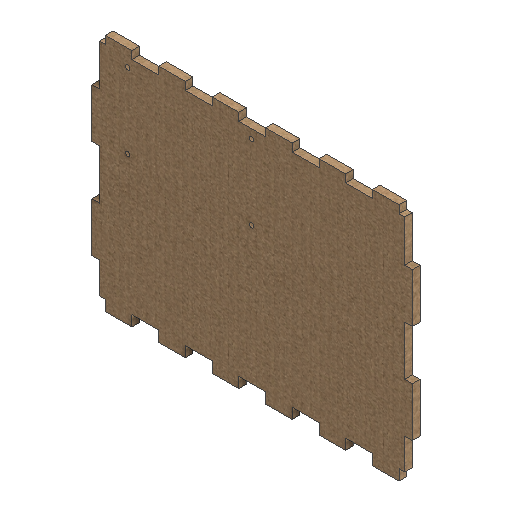
# Autodesk Inventor part: FloorPlate_1
Saved by Autodesk Inventor 2025.2 (Build 292293000, 293)
## iProperties
Created: 2025-03-07
Part Number: FloorPlate_1
Material: MDF Medium Density Fiberboard
Document SubType Name: Modeling
Designer: ahorat
Density: 0.8 g/cm^3
Appearance: Cardboard - Corrugated
Author: ahorat
Autodesk Inventor part; units mm, degrees
ref_plane "YZ Plane" through (0, 0, 0) normal (1, 0, 0) x (0, 1, 0)
ref_plane "XZ Plane" through (0, 0, 0) normal (0, 1, 0) x (-1, 0, 0)
ref_plane "XY Plane" through (0, 0, 0) normal (0, 0, 1) x (1, 0, 0)
sketch "Sketch1" plane through (0, 0, 0) normal (0, 0, 1) x (1, 0, 0)
  line L0 (-105, -80.9) -> (105, -80.9)
  line L1 (105, -80.9) -> (105, 80.9)
  line L2 (105, 80.9) -> (-105, 80.9)
  line L3 (-105, 80.9) -> (-105, -80.9)
  line L4 (-105, -80.9) -> (105, 80.9) construction
  line L5 (105, -80.9) -> (-105, 80.9) construction
  point P0 (0, 0)
  dimension "d0" = 210
  dimension "d1" = 161.8
  constraints: 12 end point, 2 midpoint, 2 parallel, 1 horizontal, 1 perpendicular
  measures "d0" distance of L1.end L2.end
  measures "d1" distance of L0.end L1.end
extrude "Extrusion1" add sketch "Sketch1" along normal blind 5
sketch "Sketch3" plane through (0, 0, 0) normal (0, 0, -1) x (-1, 0, 0)
  line L0 (0.5, 69.9) -> (81.5, 69.9)
  line L1 (81.5, 69.9) -> (81.5, 20.9)
  line L2 (81.5, 20.9) -> (0.5, 20.9)
  line L3 (0.5, 20.9) -> (0.5, 69.9)
  line L4 (105, 80.9) -> (105, -80.9) projected
  line L5 (-105, 80.9) -> (105, 80.9) projected
  point P0 (0, 0)
  dimension "d20" = 49
  dimension "d21" = 81
  dimension "d22" = 23.5
  dimension "d23" = 11
  constraints: 8 end point, 4 coincident, 2 parallel, 1 horizontal, 1 perpendicular
  measures "d20" distance of L2.end L0.start
  measures "d21" distance of L0.start L0.end
  measures "d22" distance between parallel lines of L4 L1
  measures "d23" distance between parallel lines of L5 L0
hole "Hole2" at (-0.5, 69.9, 0) at (-81.5, 69.9, 0) at (-0.5, 20.9, 0) at (-81.5, 20.9, 0) direction (0, 0, 1) diameter 3 end through all countersink diameter 4 countersink angle 90
sketch "Sketch4" plane through (0, 0, 0) normal (0, 0, -1) x (-1, 0, 0)
  line L0 (-105, 80.9) -> (105, 80.9) projected
  circle A0 centre (81.5, 20.9) radius 2 projected
  circle A1 centre (0.5, 20.9) radius 2 projected
  circle A2 centre (81.5, 69.9) radius 2 projected
  circle A3 centre (0.5, 69.9) radius 2 projected
  line L1 (-105, -80.9) -> (-105, 80.9) projected
  line L2 (105, -80.9) -> (-105, -80.9) projected
  line L3 (105, 80.9) -> (105, -80.9) projected
  line L4 (-105, 80.9) -> (105, 80.9) projected
  line L5 (8.8, 80.9) -> (-8.8, 80.9)
  line L6 (-8.8, 80.9) -> (-8.8, 75.8)
  line L7 (-8.8, 75.8) -> (8.8, 75.8)
  line L8 (8.8, 75.8) -> (8.8, 80.9)
  line L9 (-26.2, 75.8) -> (-26.2, 80.9)
  line L10 (-26.2, 80.9) -> (-43.8, 80.9)
  line L11 (-43.8, 80.9) -> (-43.8, 75.8)
  line L12 (-43.8, 75.8) -> (-26.2, 75.8)
  line L13 (-61.2, 75.8) -> (-61.2, 80.9)
  line L14 (-61.2, 80.9) -> (-78.8, 80.9)
  line L15 (-78.8, 80.9) -> (-78.8, 75.8)
  line L16 (-78.8, 75.8) -> (-61.2, 75.8)
  line L17 (-96.2, 75.8) -> (-96.2, 80.9)
  line L18 (-96.2, 80.9) -> (-113.8, 80.9)
  line L19 (-113.8, 80.9) -> (-113.8, 75.8)
  line L20 (-113.8, 75.8) -> (-96.2, 75.8)
  line L21 (26.2, 80.9) -> (26.2, 75.8)
  line L22 (43.8, 80.9) -> (26.2, 80.9)
  line L23 (43.8, 75.8) -> (43.8, 80.9)
  line L24 (26.2, 75.8) -> (43.8, 75.8)
  line L25 (61.2, 80.9) -> (61.2, 75.8)
  line L26 (78.8, 80.9) -> (61.2, 80.9)
  line L27 (78.8, 75.8) -> (78.8, 80.9)
  line L28 (61.2, 75.8) -> (78.8, 75.8)
  line L29 (96.2, 80.9) -> (96.2, 75.8)
  line L30 (113.8, 80.9) -> (96.2, 80.9)
  line L31 (113.8, 75.8) -> (113.8, 80.9)
  line L32 (96.2, 75.8) -> (113.8, 75.8)
  line L33 (0, 0) -> (105, 0) construction
  point P0 (0, 75.8)
  point P1 (8.8, 80.9)
  point P2 (-8.8, 80.9)
  point P3 (0, 80.9)
  point P4 (-35, 80.9)
  point P5 (-35, 75.8)
  point P6 (-70, 80.9)
  point P7 (-70, 75.8)
  point P8 (-105, 80.9)
  point P9 (-105, 75.8)
  point P10 (35, 75.8)
  point P11 (35, 80.9)
  point P12 (70, 75.8)
  point P13 (70, 80.9)
  point P14 (105, 75.8)
  point P15 (105, 80.9)
  point P16 (-105, 75.8)
  point P17 (105, 75.8)
  dimension "d43" = 210
  dimension "d44" = 17.6
  dimension "d45" = 5.1
  dimension "d48" = 35
  dimension "d55" = 35
  constraints: 58 end point, 3 horizontal, 3 midpoint, 2 parallel, 1 perpendicular, 1 point on line, 1 vertical alignment, 60 other
  measures "d43" distance of L0.start L0.end
  measures "d44" distance of L6.end L7.end
  measures "d45" distance of L7.end L5.start
  measures "d48" distance of L5.start L9.end
  measures "d55" distance of L6.end L21.end
extrude "Extrusion2" cut sketch "Sketch4" against normal blind 10 contours L0 L17 L20 L1 | L0 L13 L16 L15 | L0 L9 L12 L11 | L32 L29 L0 L3 | L0 L8 L7 L6 | L27 L28 L25 L0 | L0 L23 L24 L21
sketch "Sketch5" plane through (0, 0, 0) normal (0, 0, -1) x (-1, 0, 0)
  line L0 (-105, -80.9) -> (-105, 80.9) projected
  line L1 (-105, 80.9) -> (26.2, 80.9) projected
  line L2 (-105, 48.49) -> (-99.9, 48.49)
  line L3 (-99.9, 48.49) -> (-99.9, 80.9)
  line L4 (-99.9, 80.9) -> (-105, 80.9)
  line L5 (-105, 80.9) -> (-105, 48.49)
  line L6 (-105, 16.23) -> (-99.9, 16.23)
  line L7 (-99.9, 16.23) -> (-99.9, -16.23)
  line L8 (-99.9, -16.23) -> (-105, -16.23)
  line L9 (-105, -16.23) -> (-105, 16.23)
  line L10 (-105, -80.9) -> (-99.9, -80.9)
  line L11 (-99.9, -80.9) -> (-99.9, -48.49)
  line L12 (-99.9, -48.49) -> (-105, -48.49)
  line L13 (-105, -48.49) -> (-105, -80.9)
  line L14 (-102.45, 48.49) -> (-102.45, 16.23) construction
  line L15 (-102.45, -48.49) -> (-102.45, -16.23) construction
  line L16 (0, 0) -> (0, 62.5) construction
  line L17 (105, -80.9) -> (105, 80.9)
  line L18 (105, 80.9) -> (96.35, 80.9)
  line L19 (105, 48.49) -> (99.9, 48.49)
  line L20 (99.9, 48.49) -> (99.9, 80.9)
  line L21 (99.9, 80.9) -> (105, 80.9)
  line L22 (105, 80.9) -> (105, 48.49)
  line L23 (105, 16.23) -> (99.9, 16.23)
  line L24 (99.9, 16.23) -> (99.9, -16.23)
  line L25 (99.9, -16.23) -> (105, -16.23)
  line L26 (105, -16.23) -> (105, 16.23)
  line L27 (105, -80.9) -> (99.9, -80.9)
  line L28 (99.9, -80.9) -> (99.9, -48.49)
  line L29 (99.9, -48.49) -> (105, -48.49)
  line L30 (105, -48.49) -> (105, -80.9)
  line L31 (102.45, 48.49) -> (102.45, 16.23) construction
  line L32 (102.45, -48.49) -> (102.45, -16.23) construction
  point P0 (-96.35, 80.9)
  point P1 (-99.9, 0)
  point P2 (-105, 0)
  point P3 (99.9, 0)
  point P4 (105, 0)
  point P5 (-105, -48.49)
  point P6 (-105, 16.23)
  point P7 (-105, -16.23)
  dimension "d37" = 32.46
  dimension "d38" = 161.8
  dimension "d39" = 5.1
  dimension "d40" = 32.26
  constraints: 62 end point, 20 symmetric about line, 12 point on line, 6 midpoint, 6 parallel, 4 perpendicular, 3 horizontal, 1 collinear, 1 horizontal alignment, 1 vertical
  measures "d37" distance of L6.end L7.end
  measures "d38" distance of L0.start L0.end
  measures "d39" distance of L2.start L2.end
  measures "d40" distance of L14.end L14.start
extrude "Extrusion3" cut sketch "Sketch5" against normal blind 10
sketch "Sketch7" plane through (0, 0, 5) normal (0, 0, 1) x (1, 0, 0)
  line L0 (-105, -48.49) -> (105, -48.49)
  line L1 (8.8, -68.9) -> (-8.8, -68.9)
  line L2 (-8.8, -68.9) -> (-8.8, -80.9)
  line L3 (-8.8, -80.9) -> (8.8, -80.9)
  line L4 (8.8, -80.9) -> (8.8, -68.9)
  line L5 (-26.2, -80.9) -> (-26.2, -68.9)
  line L6 (-26.2, -68.9) -> (-43.8, -68.9)
  line L7 (-43.8, -68.9) -> (-43.8, -80.9)
  line L8 (-43.8, -80.9) -> (-26.2, -80.9)
  line L9 (-61.2, -80.9) -> (-61.2, -68.9)
  line L10 (-61.2, -68.9) -> (-78.8, -68.9)
  line L11 (-78.8, -68.9) -> (-78.8, -80.9)
  line L12 (-78.8, -80.9) -> (-61.2, -80.9)
  line L13 (-96.2, -80.9) -> (-96.2, -68.9)
  line L14 (-96.2, -68.9) -> (-113.8, -68.9)
  line L15 (-113.8, -68.9) -> (-113.8, -80.9)
  line L16 (-113.8, -80.9) -> (-96.2, -80.9)
  line L17 (26.2, -68.9) -> (26.2, -80.9)
  line L18 (43.8, -68.9) -> (26.2, -68.9)
  line L19 (43.8, -80.9) -> (43.8, -68.9)
  line L20 (26.2, -80.9) -> (43.8, -80.9)
  line L21 (61.2, -68.9) -> (61.2, -80.9)
  line L22 (78.8, -68.9) -> (61.2, -68.9)
  line L23 (78.8, -80.9) -> (78.8, -68.9)
  line L24 (61.2, -80.9) -> (78.8, -80.9)
  line L25 (96.2, -68.9) -> (96.2, -80.9)
  line L26 (113.8, -68.9) -> (96.2, -68.9)
  line L27 (113.8, -80.9) -> (113.8, -68.9)
  line L28 (96.2, -80.9) -> (113.8, -80.9)
  line L29 (-99.9, -80.9) -> (99.9, -80.9) projected
  point P0 (0, 0)
  point P1 (0, -80.9)
  point P2 (0, -48.49)
  point P3 (-35, -48.49)
  point P4 (-35, -80.9)
  point P5 (-70, -48.49)
  point P6 (-70, -80.9)
  point P7 (-105, -48.49)
  point P8 (-105, -80.9)
  point P9 (35, -80.9)
  point P10 (35, -48.49)
  point P11 (70, -80.9)
  point P12 (70, -48.49)
  point P13 (105, -80.9)
  point P14 (105, -48.49)
  point P15 (0, -80.9)
  point P16 (105, -48.49)
  dimension "d68" = 210
  dimension "d69" = 17.6
  dimension "d70" = 12
  dimension "d71" = 35
  dimension "d72" = 35
  constraints: 58 end point, 3 coincident, 3 horizontal, 3 midpoint, 2 parallel, 1 perpendicular, 1 vertical alignment, 60 other
  measures "d68" distance of L0.start L0.end
  measures "d69" distance of L2.end L4.start
  measures "d70" distance of L4.start L4.end
  measures "d71" distance of L4.end L6.start
  measures "d72" distance of L2.end L17.end
extrude "Extrusion4" cut sketch "Sketch7" against normal blind 10
sketch "Sketch8" plane through (0, 0, 5) normal (0, 0, 1) x (1, 0, 0)
  line L0 (-96.2, -68.9) -> (-96.2, -80.9) projected
  line L1 (-96.2, -75.9) -> (96.2, -75.9)
  line L2 (96.2, -80.9) -> (96.2, -68.9) projected
  line L3 (-96.2, -80.9) -> (-78.8, -80.9) projected
  line L4 (61.2, -80.9) -> (61.2, -68.9) projected
  line L5 (61.2, -68.9) -> (78.8, -68.9) projected
  line L6 (78.8, -68.9) -> (78.8, -80.9) projected
  line L7 (78.8, -80.9) -> (96.2, -80.9) projected
  line L8 (96.2, -80.9) -> (96.2, -68.9) projected
  line L9 (96.2, -68.9) -> (99.9, -68.9) projected
  line L10 (99.9, -68.9) -> (99.9, -48.49) projected
  line L11 (99.9, -48.49) -> (105, -48.49) projected
  line L12 (105, -48.49) -> (105, -16.23) projected
  line L13 (105, -16.23) -> (99.9, -16.23) projected
  line L14 (99.9, -16.23) -> (99.9, 16.23) projected
  line L15 (99.9, 16.23) -> (105, 16.23) projected
  line L16 (105, 16.23) -> (105, 48.49) projected
  line L17 (105, 48.49) -> (99.9, 48.49) projected
  line L18 (99.9, 48.49) -> (99.9, 75.8) projected
  line L19 (99.9, 75.8) -> (96.2, 75.8) projected
  line L20 (96.2, 75.8) -> (96.2, 80.9) projected
  line L21 (96.2, 80.9) -> (78.8, 80.9) projected
  line L22 (78.8, 80.9) -> (78.8, 75.8) projected
  line L23 (78.8, 75.8) -> (61.2, 75.8) projected
  line L24 (61.2, 75.8) -> (61.2, 80.9) projected
  line L25 (61.2, 80.9) -> (43.8, 80.9) projected
  line L26 (43.8, 80.9) -> (43.8, 75.8) projected
  line L27 (43.8, 75.8) -> (26.2, 75.8) projected
  line L28 (26.2, 75.8) -> (26.2, 80.9) projected
  line L29 (26.2, 80.9) -> (8.8, 80.9) projected
  line L30 (8.8, 80.9) -> (8.8, 75.8) projected
  line L31 (8.8, 75.8) -> (-8.8, 75.8) projected
  line L32 (-8.8, 75.8) -> (-8.8, 80.9) projected
  line L33 (-8.8, 80.9) -> (-26.2, 80.9) projected
  line L34 (-26.2, 80.9) -> (-26.2, 75.8) projected
  line L35 (-26.2, 75.8) -> (-43.8, 75.8) projected
  line L36 (-43.8, 75.8) -> (-43.8, 80.9) projected
  line L37 (-43.8, 80.9) -> (-61.2, 80.9) projected
  line L38 (-61.2, 80.9) -> (-61.2, 75.8) projected
  line L39 (-61.2, 75.8) -> (-78.8, 75.8) projected
  line L40 (-78.8, 75.8) -> (-78.8, 80.9) projected
  line L41 (-78.8, 80.9) -> (-96.2, 80.9) projected
  line L42 (-96.2, 80.9) -> (-96.2, 75.8) projected
  line L43 (-96.2, 75.8) -> (-99.9, 75.8) projected
  line L44 (-99.9, 75.8) -> (-99.9, 48.49) projected
  line L45 (-99.9, 48.49) -> (-105, 48.49) projected
  line L46 (-105, 48.49) -> (-105, 16.23) projected
  line L47 (-105, 16.23) -> (-99.9, 16.23) projected
  line L48 (-99.9, 16.23) -> (-99.9, -16.23) projected
  line L49 (-99.9, -16.23) -> (-105, -16.23) projected
  line L50 (-105, -16.23) -> (-105, -48.49) projected
  line L51 (-105, -48.49) -> (-99.9, -48.49) projected
  line L52 (-99.9, -48.49) -> (-99.9, -68.9) projected
  line L53 (-99.9, -68.9) -> (-96.2, -68.9) projected
  line L54 (-96.2, -68.9) -> (-96.2, -80.9) projected
  line L55 (-96.2, -80.9) -> (-78.8, -80.9) projected
  line L56 (-78.8, -80.9) -> (-78.8, -68.9) projected
  line L57 (-78.8, -68.9) -> (-61.2, -68.9) projected
  line L58 (-61.2, -68.9) -> (-61.2, -80.9) projected
  line L59 (-61.2, -80.9) -> (-43.8, -80.9) projected
  line L60 (-43.8, -80.9) -> (-43.8, -68.9) projected
  line L61 (-43.8, -68.9) -> (-26.2, -68.9) projected
  line L62 (-26.2, -68.9) -> (-26.2, -80.9) projected
  line L63 (-26.2, -80.9) -> (-8.8, -80.9) projected
  line L64 (-8.8, -80.9) -> (-8.8, -68.9) projected
  line L65 (-8.8, -68.9) -> (8.8, -68.9) projected
  line L66 (8.8, -68.9) -> (8.8, -80.9) projected
  line L67 (8.8, -80.9) -> (26.2, -80.9) projected
  line L68 (26.2, -80.9) -> (26.2, -68.9) projected
  line L69 (26.2, -68.9) -> (43.8, -68.9) projected
  line L70 (43.8, -68.9) -> (43.8, -80.9) projected
  line L71 (43.8, -80.9) -> (61.2, -80.9) projected
  point P0 (0, 0)
  point P1 (-78.8, -75.9)
  point P2 (78.8, -75.9)
  point P3 (-43.8, -75.9)
  point P4 (-61.2, -75.9)
  point P5 (-8.8, -75.9)
  point P6 (-26.2, -75.9)
  point P7 (61.2, -75.9)
  point P8 (43.8, -75.9)
  point P9 (26.2, -75.9)
  point P10 (8.8, -75.9)
  dimension "d77" = 5
  constraints: 2 end point, 2 point on line, 1 horizontal
  measures "d77" distance between parallel lines of L3 L1
extrude "Extrusion5" cut sketch "Sketch8" against normal blind 10 contours L1 L56 L3 L0 | L1 L60 L59 L58 | L1 L64 L63 L62 | L1 L68 L67 L66 | L68 L69 L70 L1 | L1 L4 L71 L70 | L1 L2 L7 L6
equation "\"d48\" = 0.166667 * d43"
equation "\"d55\" = 0.166667 * d43"
equation "\"d71\" = 0.166667 * d68"
equation "\"d72\" = 0.166667 * d68"
body "Solid1"
